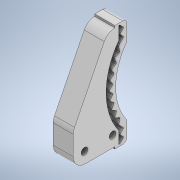
# Autodesk Inventor part: GripperClaw_silicon
Saved by Autodesk Inventor 2022.3 (Build 263350000, 350)
## iProperties
Created: 2023-06-03
Part Number: GripperClaw_silicon
Material: Generic
Document SubType Name: Modeling
Designer: komputer
Density: 1 g/cm^3
Appearance: Default
Author: komputer
Autodesk Inventor part; units mm, degrees
ref_plane "YZ Plane" through (0, 0, 0) normal (1, 0, 0) x (0, 1, 0)
ref_plane "XZ Plane" through (0, 0, 0) normal (0, 1, 0) x (-1, 0, 0)
sketch "Sketch1" plane through (0, 0, 0) normal (1, 0, 0) x (0, 1, 0)
  line L0 (-0.4351, 18.724) -> (-0.4351, -0.7378)
  arc A0 (40.6729, -0.876) -> (9.4185, -0.876) centre (25.0457, -26.3583) ccw
  line L1 (49.5732, 7.8758) -> (17.5062, 23.9101)
  line L2 (15.3569, 24.324) -> (5.1649, 24.324)
  circle A1 centre (45.9448, 4.2883) radius 1.808
  circle A2 centre (36.1506, 9.2854) radius 1.8018
  circle A3 centre (26.3531, 14.2609) radius 1.7769
  circle A4 centre (16.5584, 19.2972) radius 1.8149
  circle A5 centre (5.1645, 4.724) radius 1.7004
  circle A6 centre (5.1608, 18.7234) radius 1.7042
  line L3 (-0.4351, -0.876) -> (9.4185, -0.876)
  line L4 (40.6729, -0.876) -> (50.8969, -0.876)
  line L5 (50.8969, -0.1885) -> (50.8969, -0.876)
  line L6 (-0.4351, -0.7378) -> (-0.4351, -0.876)
  line L7 (5.529, 24.324) -> (-0.4351, 24.324)
  line L8 (-0.4351, 24.324) -> (-0.4351, 18.724)
  line L9 (15.3569, 24.324) -> (16.6785, 24.324)
  line L10 (17.5062, 23.9101) -> (16.6785, 24.324)
  line L11 (50.8969, -0.876) -> (41.3859, -0.876)
  line L12 (50.8969, 7.2139) -> (50.8969, -0.876)
  line L13 (49.5732, 7.8758) -> (50.8969, 7.2139)
  point P0 (0, 0)
  constraints: 28 end point, 7 centre point, 5 horizontal, 4 collinear, 3 vertical, 2 point on circle, 2 point on line, 1 parallel, 1 perpendicular, 8 other
extrude "Extrusion1" add sketch "Sketch1" along normal blind 10
sketch "Sketch2" plane through (10, 0, 0) normal (1, 0, 0) x (0, 0, -1)
  line L0 (-7.2139, 50.8969) -> (-24.324, 16.6785) projected
  line L1 (-24.324, 16.6785) -> (-24.324, -0.4351) projected
  line L2 (-24.324, -0.4351) -> (0.876, -0.4351) projected
  line L3 (0.876, -0.4351) -> (0.876, 9.4185) projected
  arc A0 (0.876, 40.6729) -> (0.876, 9.4185) centre (26.3583, 25.0457) ccw projected
  line L4 (0.876, 40.6729) -> (0.876, 50.8969) projected
  line L5 (0.876, 50.8969) -> (-7.2139, 50.8969) projected
  circle A1 centre (-4.724, 5.1645) radius 1.7004 projected
  circle A2 centre (-18.7234, 5.1608) radius 1.7042 projected
  circle A3 centre (-4.2883, 45.9448) radius 1.808 projected
  circle A4 centre (-9.2854, 36.1506) radius 1.8018 projected
  circle A5 centre (-19.2972, 16.5584) radius 1.8149 projected
  circle A6 centre (-14.2609, 26.3531) radius 1.7769 projected
  line L6 (-24.324, -0.4351) -> (0.876, -0.4351) projected
  line L7 (0.876, 50.8969) -> (-1.124, 50.8969)
  line L8 (-1.124, 50.8969) -> (-1.124, -0.4351)
  line L9 (-1.124, -0.4351) -> (0.876, -0.4351)
  line L10 (0.876, -0.4351) -> (0.876, 50.8969)
  line L11 (-1.124, 50.8969) -> (1.5326, 50.8969) construction
  line L12 (0.876, 40.6729) -> (0.876, 50.8969) projected
  line L13 (0.876, 48.8969) -> (3.3199, 48.8969) construction
  line L14 (-1.124, 50.8969) -> (0.876, 48.8969)
  line L15 (0.876, 48.8969) -> (-1.124, 46.8969)
  line L16 (-1.124, 46.8969) -> (0.876, 44.8969)
  line L17 (0.876, 44.8969) -> (-1.124, 42.8969)
  line L18 (-1.124, 42.8969) -> (0.876, 40.8969)
  line L19 (0.876, 40.8969) -> (-1.124, 38.8969)
  line L20 (-1.124, 38.8969) -> (0.876, 36.8969)
  line L21 (0.876, 36.8969) -> (-1.124, 34.8969)
  line L22 (-1.124, 34.8969) -> (0.876, 32.8969)
  line L23 (0.876, 32.8969) -> (-1.124, 30.8969)
  line L24 (-1.124, -0.4351) -> (0.876, 1.5649)
  line L25 (-1.124, -0.4351) -> (1.7045, -0.4351) construction
  line L26 (0.876, 1.5649) -> (-1.124, 3.5649)
  line L27 (0.876, 1.5649) -> (3.7045, 1.5649) construction
  line L28 (0.876, 5.5649) -> (-1.124, 7.5649)
  line L29 (-1.124, 3.5649) -> (0.876, 5.5649)
  line L30 (0.876, 9.5649) -> (-1.124, 11.5649)
  line L31 (-1.124, 7.5649) -> (0.876, 9.5649)
  line L32 (0.876, 13.5649) -> (-1.124, 15.5649)
  line L33 (-1.124, 11.5649) -> (0.876, 13.5649)
  line L34 (0.876, 17.5649) -> (-1.124, 19.5649)
  line L35 (-1.124, 15.5649) -> (0.876, 17.5649)
  arc A7 (0.876, 40.6729) -> (0.876, 9.4185) centre (26.3583, 25.0457) ccw projected
  line L36 (26.3583, 25.0457) -> (25.3653, 25.0457)
  line L37 (-3.5341, 25.0457) -> (-4.5271, 25.0457)
  circle A8 centre (25.3653, 25.0457) radius 29.8923
  point P0 (0, 0)
  point P1 (0.2094, 8.8984)
  point P2 (0.876, 7.9042)
  point P3 (0.876, 42.1872)
  point P4 (0.3551, 41.4178)
  dimension "d2" = 2
  dimension "d5" = 45
  dimension "d8" = 45
  dimension "d11" = 4
  dimension "d16" = 45
  dimension "d17" = 135
  dimension "d20" = 4
  dimension "d25" = 0.993
  dimension "d26" = 0.993
  constraints: 60 end point, 7 horizontal, 5 point on line, 2 equal length, 2 parallel, 2 vertical, 1 coincident, 1 perpendicular, 1 point on circle, 43 other
  measures "d2" distance of L9.end L8.end
  measures "d5" angle of L8 L14
  measures "d8" angle of L8 L15
  measures "d11" distance of L7.end L16.start
  measures "d16" angle of L25 L24
  measures "d17" angle of L27 L26
  measures "d20" distance of L24.end L28.start
  measures "d25" distance of L36.start L36.end
  measures "d26" distance of L37.start L37.end
extrude "Extrusion2" cut sketch "Sketch2" against normal blind 10 contours L5 L4 L14 | L15 L4 L16 | L24 L3 L2 | L17 L4 A8 L18 | L29 L3 L26 | L20 A0 L8 | A8 L18 L19 | L19 L4 A0 L20 | L8 A0 L37 A8 | A8 L4 L18 | A8 L3 L10 L4 | L31 A8 L3 L28 | L8 A0 | A0 L20 L21 L8 | A0 L10 L20 | L37 A0 L8 A8 | L8 L30 A0 L31 A8 | L31 A0 L3 A8 | L22 L23 L8 | L21 L10 L22 | L33 A0 L30 | L8 A0 L33 | L31 L10 A0 | A0 L30 L31 | L8 L32 L33 A0 | L23 L10 L34 L8 | A0 L33 L10 L30 | L35 L10 L32 | L8 L34 L35
sketch "Sketch3" plane through (0, 0, 0) normal (-1, 0, 0) x (0, 0, 1)
  arc A0 (-0.2094, 8.8984) -> (-0.3551, 41.4178) centre (-25.3653, 25.0457) ccw projected
  arc A1 (-0.2094, 8.8984) -> (-0.3551, 41.4178) centre (-25.3653, 25.0457) ccw projected
  line L0 (4.527, 24.9765) -> (6.527, 24.9718)
  line L1 (6.527, 24.9718) -> (4.4503, 22.9047)
  line L2 (6.527, 24.9718) -> (4.4599, 27.0485)
  line L3 (6.2269, 29.4111) -> (4.4581, 27.0751)
  line L4 (6.2269, 29.4111) -> (3.8909, 31.1799)
  line L5 (5.3119, 33.7654) -> (3.8854, 31.206)
  line L6 (5.3119, 33.7654) -> (2.7525, 35.1919)
  line L7 (3.7998, 37.95) -> (2.7434, 35.2169)
  line L8 (3.7998, 37.95) -> (1.0668, 39.0064)
  line L9 (1.7201, 41.8834) -> (1.0543, 39.0299)
  line L10 (1.7201, 41.8834) -> (-1.1334, 42.5491)
  line L11 (-0.8869, 45.4891) -> (-1.149, 42.5707)
  line L12 (-0.8869, 45.4891) -> (-3.8052, 45.7512)
  line L13 (-3.9703, 48.6968) -> (-3.8237, 45.7704)
  line L14 (-3.9703, 48.6968) -> (-6.8967, 48.5503)
  line L15 (-7.4701, 51.4443) -> (-6.9176, 48.5667)
  line L16 (-7.4701, 51.4443) -> (-10.3476, 50.8919)
  line L17 (-11.3182, 53.6779) -> (-10.3707, 50.9052)
  line L18 (-11.3182, 53.6779) -> (-14.0909, 52.7304)
  line L19 (-15.4397, 55.3542) -> (-14.1155, 52.7404)
  line L20 (-15.4397, 55.3542) -> (-18.0535, 54.03)
  line L21 (-19.7544, 56.4406) -> (-18.0794, 54.0366)
  line L22 (-19.7544, 56.4406) -> (-22.1585, 54.7656)
  line L23 (-24.1784, 56.916) -> (-22.185, 54.7684)
  line L24 (-24.1784, 56.916) -> (-26.3259, 54.9226)
  line L25 (-28.6254, 56.771) -> (-26.3526, 54.9218)
  line L26 (-28.6254, 56.771) -> (-30.4746, 54.4982)
  line L27 (-33.009, 56.0085) -> (-30.5009, 54.4936)
  line L28 (-33.009, 56.0085) -> (-34.5239, 53.5004)
  line L29 (-37.2438, 54.6434) -> (-34.5493, 53.4923)
  line L30 (-37.2438, 54.6434) -> (-38.3949, 51.9489)
  line L31 (-41.2474, 52.7022) -> (-38.4189, 51.9373)
  line L32 (-41.2474, 52.7022) -> (-42.0123, 49.8737)
  line L33 (-44.9419, 50.2227) -> (-42.0344, 49.8588)
  line L34 (-44.9419, 50.2227) -> (-45.3057, 47.3152)
  line L35 (-48.2553, 47.2531) -> (-45.3255, 47.2975)
  line L36 (-48.2553, 47.2531) -> (-48.2109, 44.3233)
  line L37 (-51.1232, 43.8513) -> (-48.2281, 44.303)
  line L38 (-51.1232, 43.8513) -> (-50.6715, 40.9562)
  line L39 (-53.4898, 40.0835) -> (-50.6857, 40.9337)
  line L40 (-53.4898, 40.0835) -> (-52.6396, 37.2794)
  line L41 (-55.3089, 36.023) -> (-52.6505, 37.2551)
  line L42 (-55.3089, 36.023) -> (-54.0767, 33.3645)
  line L43 (-56.5452, 31.7488) -> (-54.0841, 33.3389)
  line L44 (-56.5452, 31.7488) -> (-54.9551, 29.2877)
  line L45 (-57.1747, 27.3441) -> (-54.9588, 29.2613)
  line L46 (-57.1747, 27.3441) -> (-55.2575, 25.1283)
  line L47 (-57.185, 22.8948) -> (-55.2575, 25.1017)
  line L48 (-57.185, 22.8948) -> (-54.9781, 20.9673)
  line L49 (-56.5759, 18.4872) -> (-54.9744, 20.9409)
  line L50 (-56.5759, 18.4872) -> (-54.1223, 16.8857)
  line L51 (-55.3594, 14.2074) -> (-54.115, 16.8601)
  line L52 (-55.3594, 14.2074) -> (-52.7068, 12.9629)
  line L53 (-53.5591, 10.1385) -> (-52.696, 12.9385)
  line L54 (-53.5591, 10.1385) -> (-50.7591, 9.2753)
  line L55 (-51.2101, 6.3597) -> (-50.745, 9.2527)
  line L56 (-51.2101, 6.3597) -> (-48.3171, 5.8946)
  line L57 (-48.358, 2.9447) -> (-48.3, 5.8742)
  line L58 (-48.358, 2.9447) -> (-45.4284, 2.8867)
  line L59 (-45.0583, -0.0402) -> (-45.4087, 2.8689)
  line L60 (-45.0583, -0.0402) -> (-42.1492, 0.3101)
  line L61 (-41.3754, -2.5368) -> (-42.1272, 0.2952)
  line L62 (-41.3754, -2.5368) -> (-38.5434, -1.785)
  line L63 (-37.3808, -4.4966) -> (-38.5194, -1.7968)
  line L64 (-37.3808, -4.4966) -> (-34.681, -3.3579)
  line L65 (-33.1524, -5.8813) -> (-34.6557, -3.3662)
  line L66 (-33.1524, -5.8813) -> (-30.6373, -4.378)
  line L67 (-28.7724, -6.6641) -> (-30.6111, -4.3827)
  line L68 (-28.7724, -6.6641) -> (-26.491, -4.8254)
  line L69 (-24.3261, -6.8297) -> (-26.4644, -4.8264)
  line L70 (-24.3261, -6.8297) -> (-22.3228, -4.6914)
  line L71 (-19.9, -6.3748) -> (-22.2963, -4.6887)
  line L72 (-19.9, -6.3748) -> (-18.2138, -3.9786)
  line L73 (-15.5803, -5.3084) -> (-18.1879, -3.9722)
  line L74 (-15.5803, -5.3084) -> (-14.244, -2.7008)
  line L75 (-11.451, -3.6512) -> (-14.2193, -2.6909)
  line L76 (-11.451, -3.6512) -> (-10.4907, -0.883)
  line L77 (-7.5926, -1.4355) -> (-10.4675, -0.8697)
  line L78 (-7.5926, -1.4355) -> (-7.0268, 1.4395)
  line L79 (-4.0801, 1.2957) -> (-7.0058, 1.4558)
  line L80 (-4.0801, 1.2957) -> (-3.92, 4.2214)
  line L81 (-0.9819, 4.4892) -> (-3.9014, 4.2406)
  line L82 (-0.9819, 4.4892) -> (-1.2305, 7.4087)
  line L83 (1.6418, 8.0827) -> (-1.2148, 7.4302)
  line L84 (1.6418, 8.0827) -> (0.9892, 10.9393)
  line L85 (3.7397, 12.0065) -> (1.0018, 10.9628)
  line L86 (3.7397, 12.0065) -> (2.696, 14.7444)
  line L87 (5.2712, 16.184) -> (2.7052, 14.7694)
  line L88 (5.2712, 16.184) -> (3.8566, 18.75)
  line L89 (6.2063, 20.534) -> (3.8622, 18.7761)
  line L90 (6.2063, 20.534) -> (4.4484, 22.8782)
  line L91 (-0.876, 44.8969) -> (1.124, 42.8969) projected
  line L92 (1.124, 42.8969) -> (-0.3551, 41.4178) projected
  line L93 (1.124, 42.8969) -> (1.7201, 41.8834)
  circle A2 centre (14.2609, 26.3531) radius 1.7769 projected
  circle A3 centre (19.2972, 16.5584) radius 1.8149 projected
  circle A4 centre (9.2854, 36.1506) radius 1.8018 projected
  circle A5 centre (4.2883, 45.9448) radius 1.808 projected
  circle A6 centre (18.7234, 5.1608) radius 1.7042 projected
  circle A7 centre (4.724, 5.1645) radius 1.7004 projected
  line L94 (1.124, 50.8969) -> (-0.876, 48.8969) projected
  line L95 (-0.876, 48.8969) -> (1.124, 46.8969) projected
  line L96 (1.124, 46.8969) -> (-0.876, 44.8969) projected
  line L97 (-0.876, 44.8969) -> (1.124, 42.8969) projected
  line L98 (1.124, 42.8969) -> (-0.3551, 41.4178) projected
  arc A8 (-0.2094, 8.8984) -> (-0.3551, 41.4178) centre (-25.3653, 25.0457) ccw projected
  line L99 (-0.2094, 8.8984) -> (1.124, 7.5649) projected
  line L100 (1.124, 7.5649) -> (-0.876, 5.5649) projected
  line L101 (-0.876, 5.5649) -> (1.124, 3.5649) projected
  line L102 (1.124, 3.5649) -> (-0.876, 1.5649) projected
  line L103 (-0.876, 1.5649) -> (1.124, -0.4351) projected
  line L104 (24.324, -0.4351) -> (1.124, -0.4351) projected
  line L105 (24.324, 16.6785) -> (24.324, -0.4351) projected
  line L106 (7.2139, 50.8969) -> (24.324, 16.6785) projected
  line L107 (1.124, 50.8969) -> (7.2139, 50.8969) projected
  line L108 (-0.2094, 8.8984) -> (1.124, 7.5649) projected
  line L109 (1.124, 7.5649) -> (1.6418, 8.0827)
  circle A9 centre (-25.3653, 25.0457) radius 33.3266
  circle A10 centre (-25.3653, 25.0457) radius 28.5448
  line L110 (1.124, -0.4351) -> (-0.876, 1.5649) projected
  line L111 (1.124, -0.4351) -> (-4.8439, -0.4351)
  line L112 (-4.8439, -0.4351) -> (-4.8439, 49.8969)
  line L113 (-4.8439, 49.8969) -> (1.124, 49.8969)
  line L114 (1.124, 49.8969) -> (1.124, -0.4351)
  line L115 (1.124, 3.5649) -> (-0.876, 1.5649) projected
  line L116 (-0.876, 1.5649) -> (1.124, 1.5649)
  line L117 (-0.876, 1.5649) -> (-4.8439, 1.5649)
  line L118 (-4.876, -0.4351) -> (-2.3462, -0.4351)
  line L119 (-2.3462, -0.4351) -> (-2.3462, 49.8969)
  line L120 (-2.3462, 49.8969) -> (-4.876, 49.8969)
  line L121 (-4.876, 49.8969) -> (-4.876, -0.4351)
  line L122 (-0.876, 48.8969) -> (-4.876, 48.8969)
  line L123 (1.124, -0.4351) -> (1.6418, -0.4351)
  line L124 (1.6418, -0.4351) -> (1.6418, 5.5193)
  line L125 (1.6418, 5.5193) -> (1.124, 5.5193)
  line L126 (1.124, 5.5193) -> (1.124, -0.4351)
  line L127 (1.124, 50.8969) -> (1.624, 50.8969)
  line L128 (1.624, 50.8969) -> (1.624, 45.8969)
  line L129 (1.624, 45.8969) -> (1.124, 45.8969)
  line L130 (1.124, 45.8969) -> (1.124, 50.8969)
  line L131 (1.124, 50.8969) -> (-4.876, 50.8969)
  line L132 (-4.876, 50.8969) -> (-4.876, 49.8969)
  line L133 (-4.876, 49.8969) -> (1.124, 49.8969)
  line L134 (1.124, 49.8969) -> (1.124, 50.8969)
  line L135 (1.124, 1.5649) -> (1.6418, 1.5649)
  line L136 (1.6418, 1.5649) -> (1.6418, -0.4351)
  line L137 (1.6418, -0.4351) -> (1.124, -0.4351)
  line L138 (1.124, -0.4351) -> (1.124, 1.5649)
  line L139 (1.124, 50.8969) -> (1.624, 50.8969)
  line L140 (1.624, 50.8969) -> (1.624, 49.8969)
  line L141 (1.624, 49.8969) -> (1.124, 49.8969)
  line L142 (1.124, 49.8969) -> (1.124, 50.8969)
  line L143 (-0.876, 48.8969) -> (1.124, 46.8969) projected
  line L144 (1.624, 46.8969) -> (-0.876, 46.8969)
  line L145 (-0.876, 46.8969) -> (-0.876, 48.8969)
  line L146 (-0.876, 48.8969) -> (1.624, 48.8969)
  line L147 (1.624, 48.8969) -> (1.624, 46.8969)
  line L148 (-0.876, 5.5649) -> (1.124, 3.5649) projected
  line L149 (1.124, 3.5649) -> (1.6418, 3.5649)
  point P0 (0, 0)
  point P1 (1.124, 45.269)
  point P2 (1.124, 39.3284)
  point P3 (1.124, 38.9843)
  point P4 (2.7434, 35.2169)
  point P5 (2.7525, 35.1919)
  point P6 (3.8854, 31.206)
  point P7 (3.8909, 31.1799)
  point P8 (4.4581, 27.0751)
  point P9 (4.4599, 27.0485)
  point P10 (4.4503, 22.9047)
  point P11 (4.4484, 22.8782)
  point P12 (3.8622, 18.7761)
  point P13 (3.8566, 18.75)
  point P14 (2.7052, 14.7694)
  point P15 (2.696, 14.7444)
  point P16 (1.124, 11.0093)
  point P17 (1.124, 10.3495)
  point P18 (-2.3462, 41.9255)
  point P19 (-2.3462, 8.166)
  point P20 (-0.2094, 8.8984)
  point P21 (-4.3326, 50.8969)
  point P22 (-3.1599, 49.8969)
  dimension "d29" = 2
  dimension "d30" = 45
  dimension "d31" = 45
  dimension "d34" = 360
  dimension "d36" = 0.5
  constraints: 258 end point, 16 parallel, 11 perpendicular, 11 point on line, 9 horizontal, 3 point on circle, 2 coincident, 1 centre point, 229 other
  measures "d29" distance of L0.start L0.end
  measures "d30" angle of L1 L0
  measures "d31" angle of L0 L2
  measures "d36" distance of L128.end L129.end
extrude "Extrusion3" cut sketch "Sketch3" against normal blind 10 contours L114 L85 L86 A0 L87 L88 L89 L90 L1 L2 L3 L4 L5 L6 L7 L8 L9 L93 A9 L125 L109 L84 | L114 A9 L101 L100 | L125 A9 L114 | A9 L114 L101 | A9 L124 L149 L114 | L114 L91 L96 A9 | A9 L96 L114
extrude "Extrusion4" add sketch "Sketch3" against normal blind 10 contours L99 L100 L101 A9 L117 L119 A10 L114 A0 | L114 A10 A0 | L101 L102 L117 A9 | A10 L119 L122 A9 L145 L144 L96 L91 L92 A0 L114 | L117 L103 L111 L119 A9 | A9 L119 L117 | A9 L144 L96 | L119 A9 L122 | L131 L94 L113 A9 | L144 A9 L145 L95 | L144 L145 A9 | L119 L113 L94 L122 A9 | L122 L145 A9
sketch "Sketch4" plane through (0, 0, 0) normal (-1, 0, 0) x (0, 0, 1)
  line L0 (-2.3462, -0.4351) -> (24.324, -0.4351) projected
  line L1 (24.324, 16.6785) -> (24.324, -0.4351) projected
  line L2 (7.2139, 50.8969) -> (24.324, 16.6785) projected
  line L3 (-4.3326, 50.8969) -> (7.2139, 50.8969) projected
  arc A0 (-3.1599, 49.8969) -> (-4.3326, 50.8969) centre (-25.3653, 25.0457) ccw projected
  line L4 (-3.1599, 49.8969) -> (-2.3462, 49.8969) projected
  line L5 (-2.3462, 49.8969) -> (-2.3462, 41.9255) projected
  arc A1 (-2.3462, 8.166) -> (-2.3462, 41.9255) centre (-25.3653, 25.0457) ccw projected
  line L6 (-2.3462, 8.166) -> (-2.3462, -0.4351) projected
  circle A2 centre (14.2609, 26.3531) radius 1.7769 projected
  circle A3 centre (19.2972, 16.5584) radius 1.8149 projected
  circle A4 centre (9.2854, 36.1506) radius 1.8018 projected
  circle A5 centre (4.2883, 45.9448) radius 1.808 projected
  circle A6 centre (18.7234, 5.1608) radius 1.7042 projected
  circle A7 centre (4.724, 5.1645) radius 1.7004 projected
  line L7 (3.7397, 12.0065) -> (2.696, 14.7444) projected
  arc A8 (2.696, 14.7444) -> (2.7052, 14.7694) centre (-25.3653, 25.0457) ccw projected
  line L8 (2.7052, 14.7694) -> (5.2712, 16.184) projected
  line L9 (5.2712, 16.184) -> (3.8566, 18.75) projected
  arc A9 (3.8566, 18.75) -> (3.8622, 18.7761) centre (-25.3653, 25.0457) ccw projected
  line L10 (3.8622, 18.7761) -> (6.2063, 20.534) projected
  line L11 (6.2063, 20.534) -> (4.4484, 22.8782) projected
  arc A10 (4.4484, 22.8782) -> (4.4503, 22.9047) centre (-25.3653, 25.0457) ccw projected
  line L12 (4.4503, 22.9047) -> (6.527, 24.9718) projected
  line L13 (6.527, 24.9718) -> (4.4599, 27.0485) projected
  arc A11 (4.4599, 27.0485) -> (4.4581, 27.0751) centre (-25.3653, 25.0457) ccw projected
  line L14 (4.4581, 27.0751) -> (6.2269, 29.4111) projected
  line L15 (6.2269, 29.4111) -> (3.8909, 31.1799) projected
  arc A12 (3.8909, 31.1799) -> (3.8854, 31.206) centre (-25.3653, 25.0457) ccw projected
  line L16 (3.8854, 31.206) -> (5.3119, 33.7654) projected
  line L17 (5.3119, 33.7654) -> (2.7525, 35.1919) projected
  arc A13 (2.7525, 35.1919) -> (2.7434, 35.2169) centre (-25.3653, 25.0457) ccw projected
  line L18 (2.7434, 35.2169) -> (3.7998, 37.95) projected
  line L19 (3.7998, 37.95) -> (1.124, 38.9843) projected
  line L20 (1.124, 38.9843) -> (1.124, 39.3284) projected
  line L21 (1.124, 39.3284) -> (1.7201, 41.8834) projected
  line L22 (1.7201, 41.8834) -> (1.124, 42.8969) projected
  line L23 (1.124, 42.8969) -> (-0.876, 44.8969) projected
  line L24 (-0.876, 44.8969) -> (1.124, 46.8969) projected
  line L25 (1.124, 46.8969) -> (1.124, 45.269) projected
  arc A14 (1.6418, 5.5193) -> (1.124, 45.269) centre (-25.3653, 25.0457) ccw projected
  line L26 (1.6418, 5.5193) -> (1.6418, 3.5649) projected
  line L27 (1.6418, 3.5649) -> (1.124, 3.5649) projected
  line L28 (1.124, 3.5649) -> (-0.876, 5.5649) projected
  line L29 (-0.876, 5.5649) -> (1.6418, 8.0827) projected
  line L30 (1.6418, 8.0827) -> (1.124, 10.3495) projected
  line L31 (1.124, 10.3495) -> (1.124, 11.0093) projected
  line L32 (1.124, 11.0093) -> (3.7397, 12.0065) projected
  line L33 (-0.876, 5.5649) -> (1.124, 3.5649) projected
  line L34 (1.124, 3.5649) -> (-0.876, 1.5649)
  line L35 (1.124, 3.5649) -> (3.9524, 3.5649) construction
  line L36 (-0.876, 1.5649) -> (1.124, -0.4351)
  line L37 (1.124, -0.4351) -> (1.6418, -0.4351)
  line L38 (24.324, -0.4351) -> (-2.3462, -0.4351) projected
  line L39 (1.124, 3.5649) -> (1.6418, 3.5649) projected
  line L40 (1.6418, 3.5649) -> (1.6418, -0.4351)
  line L41 (1.124, 46.8969) -> (1.124, 50.8969)
  line L42 (-0.876, 44.8969) -> (1.124, 46.8969) projected
  line L43 (1.124, 46.8969) -> (-0.876, 48.8969)
  line L44 (1.124, 46.8969) -> (3.9524, 46.8969) construction
  line L45 (-0.876, 48.8969) -> (1.124, 50.8969)
  line L46 (1.6418, -0.4351) -> (1.124, -0.4351)
  line L47 (1.124, -0.4351) -> (1.124, 50.8969)
  line L48 (1.124, 50.8969) -> (1.6418, 50.8969)
  line L49 (1.6418, 50.8969) -> (1.6418, -0.4351)
  point P0 (0, 0)
  point P1 (1.6418, 44.5722)
  dimension "d41" = 135
  dimension "d42" = 135
  constraints: 26 end point, 4 perpendicular, 3 horizontal, 2 equal length, 2 parallel, 2 point on line, 1 vertical
  measures "d41" angle of L34 L35
  measures "d42" angle of L44 L43
extrude "Extrusion5" cut sketch "Sketch4" against normal blind 10 contours L47 L27 L40 L0 | L36 L34 L47 | A14 L25 L41 L3 L49 | L41 L43 L45
sketch "Sketch5" plane through (0, 0, 0) normal (-1, 0, 0) x (0, 0, 1)
  line L0 (-0.876, 1.5649) -> (1.124, 3.5649) projected
  line L1 (1.124, 3.5649) -> (-0.876, 5.5649) projected
  line L2 (-0.876, 5.5649) -> (1.6418, 8.0827) projected
  line L3 (1.6418, 8.0827) -> (1.124, 10.3495) projected
  line L4 (1.124, 10.3495) -> (1.124, 11.0093) projected
  line L5 (1.124, 11.0093) -> (3.7397, 12.0065) projected
  line L6 (3.7397, 12.0065) -> (2.696, 14.7444) projected
  arc A0 (2.696, 14.7444) -> (2.7052, 14.7694) centre (-25.3653, 25.0457) ccw projected
  line L7 (2.7052, 14.7694) -> (5.2712, 16.184) projected
  line L8 (5.2712, 16.184) -> (3.8566, 18.75) projected
  arc A1 (3.8566, 18.75) -> (3.8622, 18.7761) centre (-25.3653, 25.0457) ccw projected
  line L9 (3.8622, 18.7761) -> (6.2063, 20.534) projected
  line L10 (6.2063, 20.534) -> (4.4484, 22.8782) projected
  arc A2 (4.4484, 22.8782) -> (4.4503, 22.9047) centre (-25.3653, 25.0457) ccw projected
  line L11 (4.4503, 22.9047) -> (6.527, 24.9718) projected
  line L12 (6.527, 24.9718) -> (4.4599, 27.0485) projected
  arc A3 (4.4599, 27.0485) -> (4.4581, 27.0751) centre (-25.3653, 25.0457) ccw projected
  line L13 (4.4581, 27.0751) -> (6.2269, 29.4111) projected
  line L14 (6.2269, 29.4111) -> (3.8909, 31.1799) projected
  arc A4 (3.8909, 31.1799) -> (3.8854, 31.206) centre (-25.3653, 25.0457) ccw projected
  line L15 (3.8854, 31.206) -> (5.3119, 33.7654) projected
  line L16 (5.3119, 33.7654) -> (2.7525, 35.1919) projected
  arc A5 (2.7525, 35.1919) -> (2.7434, 35.2169) centre (-25.3653, 25.0457) ccw projected
  line L17 (2.7434, 35.2169) -> (3.7998, 37.95) projected
  line L18 (3.7998, 37.95) -> (1.124, 38.9843) projected
  line L19 (1.124, 38.9843) -> (1.124, 39.3284) projected
  line L20 (1.124, 39.3284) -> (1.7201, 41.8834) projected
  line L21 (1.7201, 41.8834) -> (1.124, 42.8969) projected
  line L22 (1.124, 42.8969) -> (-0.876, 44.8969) projected
  line L23 (-0.876, 44.8969) -> (1.124, 46.8969) projected
  line L24 (1.124, 46.8969) -> (-0.876, 48.8969) projected
  line L25 (-0.876, 48.8969) -> (1.124, 50.8969) projected
  line L26 (-4.3326, 50.8969) -> (1.124, 50.8969) projected
  arc A6 (-3.1599, 49.8969) -> (-4.3326, 50.8969) centre (-25.3653, 25.0457) ccw projected
  line L27 (-3.1599, 49.8969) -> (-2.3462, 49.8969) projected
  line L28 (-2.3462, 49.8969) -> (-2.3462, 41.9255) projected
  arc A7 (-2.3462, 8.166) -> (-2.3462, 41.9255) centre (-25.3653, 25.0457) ccw projected
  line L29 (-2.3462, 8.166) -> (-2.3462, -0.4351) projected
  line L30 (-2.3462, -0.4351) -> (1.124, -0.4351) projected
  line L31 (1.124, -0.4351) -> (-0.876, 1.5649) projected
  line L32 (-3.1599, 49.8969) -> (-2.3462, 49.8969) projected
  line L33 (-2.3462, 49.8969) -> (-5.8456, 49.8969)
  line L34 (-5.8456, 49.8969) -> (-5.8456, 51.8665)
  line L35 (-5.8456, 51.8665) -> (-2.3462, 51.8665)
  line L36 (-2.3462, 51.8665) -> (-2.3462, 49.8969)
  point P0 (0, 0)
  point P1 (-3.1599, 49.8969)
  constraints: 8 end point, 2 parallel, 1 horizontal, 1 perpendicular
extrude "Extrusion6" cut sketch "Sketch5" against normal blind 10 contours L27 A6 L26 L36 | L33 L34 L35 L36 L26 A6
sketch "Sketch6" plane through (0, 0, 0) normal (-1, 0, 0) x (0, 0, 1)
  circle A0 centre (4.724, 5.1645) radius 1.7004 projected
  circle A1 centre (18.7234, 5.1608) radius 1.7042 projected
  circle A2 centre (4.2883, 45.9448) radius 1.808 projected
  circle A3 centre (9.2854, 36.1506) radius 1.8018 projected
  circle A4 centre (19.2972, 16.5584) radius 1.8149 projected
  circle A5 centre (14.2609, 26.3531) radius 1.7769 projected
  line L0 (1.6418, 5.5193) -> (1.6418, -0.4351) projected
  line L1 (1.6418, -0.4351) -> (24.324, -0.4351) projected
  line L2 (24.324, 16.6785) -> (24.324, -0.4351) projected
  line L3 (7.2139, 50.8969) -> (24.324, 16.6785) projected
  line L4 (1.6418, 50.8969) -> (7.2139, 50.8969) projected
  line L5 (1.6418, 50.8969) -> (1.6418, 44.5722) projected
  arc A6 (1.6418, 5.5193) -> (1.6418, 44.5722) centre (-25.3653, 25.0457) ccw projected
  line L6 (-2.3462, 50.8969) -> (-2.3462, 41.9255) projected
  arc A7 (-2.3462, 8.166) -> (-2.3462, 41.9255) centre (-25.3653, 25.0457) ccw projected
  line L7 (-2.3462, 8.166) -> (-2.3462, -0.4351) projected
  line L8 (-2.3462, -0.4351) -> (1.124, -0.4351) projected
  line L9 (1.124, -0.4351) -> (-0.876, 1.5649) projected
  line L10 (-0.876, 1.5649) -> (1.124, 3.5649) projected
  line L11 (1.124, 3.5649) -> (-0.876, 5.5649) projected
  line L12 (-0.876, 5.5649) -> (1.6418, 8.0827) projected
  line L13 (1.6418, 8.0827) -> (1.124, 10.3495) projected
  line L14 (1.124, 10.3495) -> (1.124, 11.0093) projected
  line L15 (1.124, 11.0093) -> (3.7397, 12.0065) projected
  line L16 (3.7397, 12.0065) -> (2.696, 14.7444) projected
  arc A8 (2.696, 14.7444) -> (2.7052, 14.7694) centre (-25.3653, 25.0457) ccw projected
  line L17 (2.7052, 14.7694) -> (5.2712, 16.184) projected
  line L18 (5.2712, 16.184) -> (3.8566, 18.75) projected
  arc A9 (3.8566, 18.75) -> (3.8622, 18.7761) centre (-25.3653, 25.0457) ccw projected
  line L19 (3.8622, 18.7761) -> (6.2063, 20.534) projected
  line L20 (6.2063, 20.534) -> (4.4484, 22.8782) projected
  arc A10 (4.4484, 22.8782) -> (4.4503, 22.9047) centre (-25.3653, 25.0457) ccw projected
  line L21 (4.4503, 22.9047) -> (6.527, 24.9718) projected
  line L22 (6.527, 24.9718) -> (4.4599, 27.0485) projected
  arc A11 (4.4599, 27.0485) -> (4.4581, 27.0751) centre (-25.3653, 25.0457) ccw projected
  line L23 (4.4581, 27.0751) -> (6.2269, 29.4111) projected
  line L24 (6.2269, 29.4111) -> (3.8909, 31.1799) projected
  arc A12 (3.8909, 31.1799) -> (3.8854, 31.206) centre (-25.3653, 25.0457) ccw projected
  line L25 (3.8854, 31.206) -> (5.3119, 33.7654) projected
  line L26 (5.3119, 33.7654) -> (2.7525, 35.1919) projected
  arc A13 (2.7525, 35.1919) -> (2.7434, 35.2169) centre (-25.3653, 25.0457) ccw projected
  line L27 (2.7434, 35.2169) -> (3.7998, 37.95) projected
  line L28 (3.7998, 37.95) -> (1.124, 38.9843) projected
  line L29 (1.124, 38.9843) -> (1.124, 39.3284) projected
  line L30 (1.124, 39.3284) -> (1.7201, 41.8834) projected
  line L31 (1.7201, 41.8834) -> (1.124, 42.8969) projected
  line L32 (1.124, 42.8969) -> (-0.876, 44.8969) projected
  line L33 (-0.876, 44.8969) -> (1.124, 46.8969) projected
  line L34 (1.124, 46.8969) -> (-0.876, 48.8969) projected
  line L35 (-0.876, 48.8969) -> (1.124, 50.8969) projected
  line L36 (-2.3462, 50.8969) -> (1.124, 50.8969) projected
  line L37 (-2.3462, -0.4351) -> (-2.3462, 8.166) projected
  line L38 (-2.3462, -0.4351) -> (3.6538, -0.4351)
  line L39 (3.6538, -0.4351) -> (3.6538, -1.4351)
  line L40 (3.6538, -1.4351) -> (-2.3462, -1.4351)
  line L41 (-2.3462, -1.4351) -> (-2.3462, -0.4351)
  line L42 (-2.3462, 50.8969) -> (3.6538, 50.8969)
  line L43 (3.6538, 50.8969) -> (3.6538, 51.8969)
  line L44 (3.6538, 51.8969) -> (-2.3462, 51.8969)
  line L45 (-2.3462, 51.8969) -> (-2.3462, 50.8969)
  point P0 (0, 0)
  dimension "d47" = 6
  dimension "d48" = 1
  dimension "d49" = 6
  dimension "d50" = 1
  constraints: 16 end point, 4 parallel, 2 horizontal, 2 perpendicular
  measures "d47" distance of L39.end L40.end
  measures "d48" distance of L38.end L39.end
  measures "d49" distance of L44.end L43.end
  measures "d50" distance of L43.end L42.end
extrude "Extrusion7" add sketch "Sketch6" against normal blind 10 contours L1 L39 L40 L41 L8 L38 | L42 L36 L45 L44 L43 L4
ref_plane "Work Plane1" through (5, 0, 0) normal (-1, 0, 0) x (0, 0, 1)
sketch "Sketch7" plane through (0, 0, 0) normal (-1, 0, 0) x (0, 0, 1)
  circle A0 centre (19.2972, 16.5584) radius 1.8149 projected
  circle A1 centre (14.2609, 26.3531) radius 1.7769 projected
  circle A2 centre (9.2854, 36.1506) radius 1.8018 projected
  circle A3 centre (4.2883, 45.9448) radius 1.808 projected
  point P0 (0, 0)
extrude "Extrusion8" add sketch "Sketch7" against normal blind 10
sketch "Sketch8" plane through (5, 0, 0) normal (-1, 0, 0) x (0, 0, 1)
  arc A0 (1.6418, 5.5193) -> (1.6418, 44.5722) centre (-25.3653, 25.0457) ccw projected
  arc A1 (1.6418, 5.5193) -> (1.6418, 44.5722) centre (-25.3653, 25.0457) ccw projected
  line L0 (7.9613, 25.0457) -> (10.9613, 25.0457)
  circle A2 centre (-25.3653, 25.0457) radius 36.3266
  line L1 (6.8673, 8.2921) -> (5.2777, 12.6845)
  line L2 (3.757, 41.2493) -> (4.6037, 45.5757)
  point P0 (0, 0)
  point P1 (5.4219, 12.286)
  dimension "d55" = 3
  constraints: 6 end point, 6 point on circle, 1 centre point, 1 coincident, 1 horizontal
  measures "d55" distance of L0.start L0.end
extrude "Extrusion9" cut sketch "Sketch8" along normal mid plane 6 contours L0 A2 L1 A0 | A0 L2 A2 L0
fillet "Fillet1" radius 0.5 14 edges at (5, 37.95, 3.7998) (5, 41.8834, 1.7201) (5, 42.8969, 1.124) (5, 46.8969, 1.124) (5, 33.7654, 5.3119) (5, 29.4111, 6.2269) (5, 24.9718, 6.527) (5, 20.534, 6.2063) (5, 16.184, 5.2712) (5, 12.0065, 3.7397) (5, 8.0827, 1.6418) (5, 3.5649, 1.124) (5, 12.286, 5.4219) (5, 41.2493, 3.757)
fillet "Fillet2" radius 0.5 21 edges at (5, 18.7761, 3.8622) (5, 22.8782, 4.4484) (5, 27.0485, 4.4599) (5, 31.1799, 3.8909) (5, 35.1919, 2.7525) (5, 38.9843, 1.124) (5, 44.8969, -0.876) (5, 48.8969, -0.876) (5, 14.7694, 2.7052) (5, 11.0093, 1.124) (5, 10.3495, 1.124) (5, 5.5649, -0.876) (5, 1.5649, -0.876) (5, 14.7444, 2.696) (5, 18.75, 3.8566) (5, 22.9047, 4.4503) (5, 27.0751, 4.4581) (5, 31.206, 3.8854) (5, 35.2169, 2.7434) (5, 8.166, -2.3462) (5, 41.9255, -2.3462)
fillet "Fillet3" radius 2 2 edges at (5, -1.4351, -2.3462) (5, 51.8969, -2.3462)
fillet "Fillet4" radius 6 3 edges at (5, 50.8969, 7.2139) (5, -0.4351, 24.324) (5, 16.6785, 24.324)
body "Solid1"
